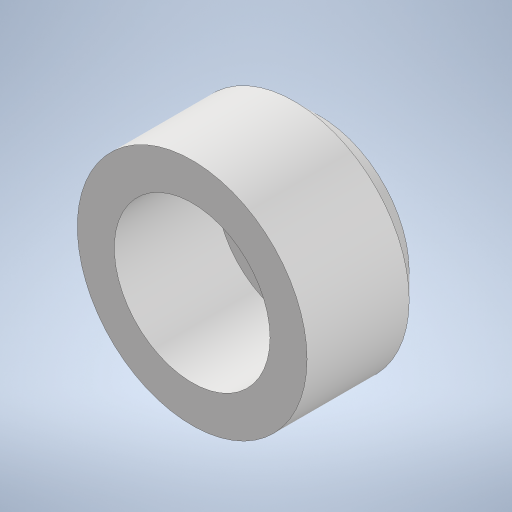
# Autodesk Inventor part: laser_diode_lid
Saved by Autodesk Inventor 2024.1 (Build 281209000, 209)
## iProperties
Created: 2023-10-07
Part Number: laser_diode_lid
Material: Generic
Document SubType Name: Modeling
Designer: l1534
Density: 1 g/cm^3
Appearance: Default
Author: l1534
Autodesk Inventor part; units mm, degrees
ref_plane "YZ Plane" through (0, 0, 0) normal (1, 0, 0) x (0, 1, 0)
ref_plane "XZ Plane" through (0, 0, 0) normal (0, 1, 0) x (-1, 0, 0)
ref_plane "XY Plane" through (0, 0, 0) normal (0, 0, 1) x (1, 0, 0)
sketch "Sketch1" plane through (0, 0, 0) normal (0, 0, 1) x (1, 0, 0)
  circle A0 centre (0, 0) radius 4.5
  dimension "d0" = 9
  constraints: 1 centre point, 1 coincident
  measures "d0" diameter of A0
extrude "Extrusion1" add sketch "Sketch1" along normal blind 5
sketch "Sketch2" plane through (0, 0, 5) normal (0, 0, 1) x (1, 0, 0)
  circle A0 centre (0, 0) radius 3.05
  dimension "d3" = 6.1
  constraints: 1 centre point, 1 coincident
  measures "d3" diameter of A0
extrude "Extrusion2" cut sketch "Sketch2" against normal blind 4
chamfer "Chamfer1" distance 1 angle 45 1 edges at (-4.5, 0, 0)
sketch "Sketch3" plane through (0, 0, 1) normal (0, 0, 1) x (1, 0, 0)
  circle A0 centre (0, 0) radius 0.25
  dimension "d9" = 0.5
  constraints: 1 centre point, 1 coincident
  measures "d9" diameter of A0
extrude "Extrusion3" cut sketch "Sketch3" against normal through all
fillet "Fillet1" radius 0.5 1 edges at (-0.25, 0, 1)
body "Solid1"
